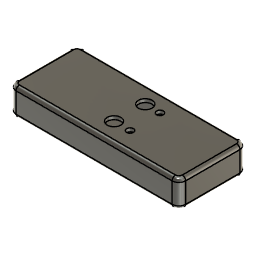
Final Exam Part 2 (Assembly) (Autodesk Fusion 360 archive; units mm, degrees)
design "Final Exam Part 2"
part number: 2026-04-19-10-33-35-140
Autodesk Fusion 360 part; units mm, degrees
sketch "Sketch1" plane through (0, 0, 0) normal (0, 0, 1) x (1, 0, 0)
  line L0 (-50, 50) -> (200, 50)
  line L1 (200, 50) -> (200, -50)
  line L2 (200, -50) -> (-50, -50)
  line L3 (-50, -50) -> (-50, 50)
  constraint horizontal L0
  constraint vertical L1
  constraint horizontal L2
  constraint vertical L3
extrude "Extrude1" add sketch "Sketch1" along normal blind 40
fillet "Fillet1" radius 10 4 edges at (-50, 50, 20) (-50, -50, 20) (200, -50, 20) (200, 50, 20)
fillet "Fillet2" radius 5 1 faces at (113.3333, -16.6667, 40)
fillet "Fillet3" radius 5 1 faces at (113.3333, -16.6667, 0)
shell "Shell1" thickness 5 removed faces 0 bodies 1
hole "Hole1" at (-50, 0, 20) direction (1, 0, 0) diameter 20.2 depth 5 tip angle 118
hole "Hole2" at (76.1159, -21.7133, 40) direction (0, 0, -1) diameter 20 depth 5 tip angle 118
hole "Hole3" at (77.3642, 23.0742, 40) direction (0, 0, -1) diameter 20.2 depth 5 tip angle 118
hole "Hole4" at (99.2532, 22.836, 40) direction (0, 0, -1) diameter 10 depth 5 tip angle 118
hole "Hole5" at (99.791, -21.8395, 40) direction (0, 0, -1) diameter 10 depth 5 tip angle 118
